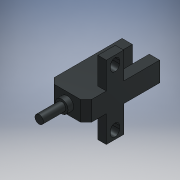
# Autodesk Inventor part: RX672-NW
Saved by Autodesk Inventor 2017 (Build 210142000, 142)
## iProperties
Part Number: RX672-NW
Material: SS41
Document SubType Name: Modeling
Designer: G
Density: 7.85 g/cm^3
Appearance: 鐵灰色
Author: G
Autodesk Inventor part; units mm, degrees
ref_plane "YZ Plane" through (0, 0, 0) normal (1, 0, 0) x (0, 1, 0)
ref_plane "XZ Plane" through (0, 0, 0) normal (0, 1, 0) x (-1, 0, 0)
ref_plane "XY Plane" through (0, 0, 0) normal (0, 0, 1) x (1, 0, 0)
sketch "草圖1" plane through (0, 0, 0) normal (0, 0, 1) x (1, 0, 0)
  line L0 (-6.7, 26.2) -> (-3, 26.2)
  line L1 (-3, 26.2) -> (-3, 17.2)
  line L2 (-3, 17.2) -> (3, 17.2)
  line L3 (3, 17.2) -> (3, 26.2)
  line L4 (3, 26.2) -> (6.7, 26.2)
  line L5 (6.7, 26.2) -> (6.7, 2)
  line L6 (-6.7, 2) -> (-6.7, 26.2)
  line L7 (-6.7, 2) -> (-4.7, 0)
  line L8 (-4.7, 0) -> (-1.5, 0)
  line L9 (6.7, 2) -> (4.7, 0)
  line L10 (4.7, 0) -> (1.5, 0)
  line L11 (-1.5, 0) -> (1.5, 0)
  point P0 (0, 0)
  point P1 (0, 17.2)
  point P2 (0, 0)
  point P3 (0, 0)
  dimension "d0" = 6
  dimension "d1" = 13.4
  dimension "d5" = 9
  dimension "d10" = 26.2
  dimension "d11" = 135
  dimension "d13" = 2
  constraints: 24 end point, 4 perpendicular, 3 coincident, 3 collinear, 2 horizontal, 2 midpoint, 2 point on line, 1 horizontal alignment, 1 vertical alignment
  measures "d0" distance of L1.end L2.end
  measures "d1" distance between parallel lines of L5 L6
  measures "d5" distance of L0.end L1.end
  measures "d10" distance between parallel lines of L0 L8
  measures "d11" angle of L8 L7
  measures "d13" horizontal distance of L6.start L7.end
extrude "擠出1" add sketch "草圖1" along normal mid plane 7
sketch "草圖2" plane through (0, 0, 0) normal (0, 0, 1) x (1, 0, 0)
  line L0 (0, 0) -> (2.3, 0)
  line L1 (1.5, -2) -> (1.5, -10)
  line L2 (1.5, -10) -> (0, -10)
  line L3 (0, -10) -> (0, 0)
  line L4 (-4.7, 0) -> (4.7, 0) construction
  line L5 (2.3, 0) -> (2.3, -2)
  line L6 (2.3, -2) -> (1.5, -2)
  point P0 (1.5, 0)
  dimension "d20" = 4.6
  dimension "d21" = 3
  dimension "d22" = 2
  dimension "d23" = 10
  constraints: 12 end point, 2 parallel, 2 perpendicular, 1 horizontal, 1 midpoint, 1 point on line, 1 vertical
  measures "d20" diameter of L5 L3
  measures "d21" diameter of L1 L3
  measures "d22" distance of L0.end L5.end
  measures "d23" distance of L2.end L0.start
revolve "迴轉1" add sketch "草圖2" angle 360 about axis through (0, -10, 0) along (0, 1, 0)
sketch "草圖3" plane through (6.7, 2, 3.5) normal (1, 0, 0) x (0, 0, -1)
  line L0 (-9.5, 11.4) -> (16.5, 11.4)
  line L1 (16.5, 11.4) -> (16.5, 5.2)
  line L2 (16.5, 5.2) -> (-9.5, 5.2)
  line L3 (-9.5, 5.2) -> (-9.5, 11.4)
  line L4 (-8.7, 8.3) -> (-4.4, 8.3) construction
  line L5 (-7.1, 6.7) -> (-6, 6.7)
  line L6 (-6, 9.9) -> (-7.1, 9.9)
  arc A0 (-7.1, 9.9) -> (-7.1, 6.7) centre (-7.1, 8.3) ccw
  arc A1 (-6, 6.7) -> (-6, 9.9) centre (-6, 8.3) ccw
  line L7 (11.4, 8.3) -> (15.7, 8.3) construction
  line L8 (13, 6.7) -> (14.1, 6.7)
  line L9 (14.1, 9.9) -> (13, 9.9)
  arc A2 (13, 9.9) -> (13, 6.7) centre (13, 8.3) ccw
  arc A3 (14.1, 6.7) -> (14.1, 9.9) centre (14.1, 8.3) ccw
  line L10 (0, -2) -> (7, -2) projected
  line L11 (-4.4, 8.3) -> (11.4, 8.3) construction
  point P0 (3.5, -2)
  point P1 (3.5, 5.2)
  point P2 (16.5, 8.3)
  point P3 (3.5, 8.3)
  dimension "d24" = 26
  dimension "d25" = 6.2
  dimension "d26" = 1.1
  dimension "d27" = 4.3
  dimension "d28" = 19
  dimension "d29" = 10.3
  constraints: 22 end point, 13 point on circle, 10 point on line, 8 tangent, 4 centre point, 4 parallel, 3 midpoint, 2 collinear, 2 horizontal, 2 perpendicular, 2 vertical alignment, 1 horizontal alignment
  measures "d24" distance of L0.start L0.end
  measures "d25" distance of L0.end L1.end
  measures "d26" distance of L9.start L9.end
  measures "d27" distance of L7.start L7.end
  measures "d28" distance of A2.centre A1.centre
  measures "d29" distance between parallel lines of L4 L10
extrude "擠出2" add sketch "草圖3" against normal blind 3
